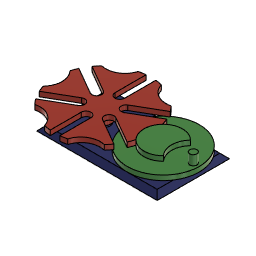
Snowflake (Autodesk Fusion 360 design; units mm, degrees)
Autodesk Fusion 360 part; units mm, degrees
note: some values were not read from the file. Set by a fixed rule: which face or edge a step refers to.
sketch "Base" plane through (0, 0, 0) normal (0, 0, 1) x (1, 0, 0) in component "Base"
  line L0 (125, 75) -> (-125, 75)
  line L1 (-125, 75) -> (-125, -75)
  line L2 (-125, -75) -> (125, -75)
  line L3 (125, -75) -> (125, 75)
  line L4 (125, 75) -> (-125, -75) construction
  line L5 (-125, 75) -> (125, -75) construction
  dimension "d1" = 250
  dimension "d2" = 150
  constraint horizontal L0
  constraint perpendicular L0 L1
  constraint parallel L0 L2
  constraint parallel L1 L3
  constraint coincident L4 origin
  constraint coincident L5 origin
  measures "d1" distance of L1.end L2.end
  measures "d2" distance of L0.end L1.end
extrude "Extrude1" add sketch "Base" along normal blind 10 makes body 1 in component "Base"
sketch "Wheels" plane through (0, 0, 10) normal (0, 0, 1) x (-1, 0, 0) in component "Base"
  line L0 (-125, 75) -> (-125, -75)
  line L1 (-125, -75) -> (125, -75)
  line L2 (125, -75) -> (125, 75)
  line L3 (125, 75) -> (-125, 75)
  line L4 (0, 0) -> (-125, 0) construction
  line L5 (0, 0) -> (125, 0) construction
  line L6 (0, -75) -> (0, 75) construction
  circle A0 centre (-62.5, 0) radius 75
  circle A1 centre (62.5, 0) radius 75
  circle A2 centre (-62.5, 0) radius 15
  circle A3 centre (62.5, 0) radius 15
  dimension "d5" = 150
  dimension "d6" = 30
  dimension "d7" = 30
  constraint coincident L4.start L5.start
  constraint midpoint L0 L4.end
  constraint midpoint L2 L5.end
  constraint midpoint L1 L6.start
  constraint midpoint L3 L6.end
  constraint midpoint L4 A0.centre
  constraint symmetric L6 A0 A1
  constraint concentric A0 A2
  constraint concentric A1 A3
  measures "d5" diameter of A0
  measures "d6" diameter of A2
  measures "d7" diameter of A3
extrude "Extrude2" add sketch "Wheels" along normal blind 20 and the other way blind -10 separate body contours L0 A0 A1 | L0 A0 | A0 A1 makes body 2 in component "Base"
copy_body "CutPasteBodies1" bodies 2 removing the originals makes body 3 in component "Crank"
extrude "Extrude3" add sketch "Wheels" along normal blind 10 contours A2 bodies 1 in component "Base"
extrude "Extrude1'" add sketch "Wheels" along normal blind 30 and the other way blind -20 separate body contours L2 A0 A1 | A0 A1 | L2 A1 makes body 4 in component "Snowflake"
extrude "Extrude4" add sketch "Wheels" along normal blind 20 contours A3 bodies 1 in component "Base"
move_face "OffsetFaces1" offset 25 1 faces at (12.1273, -7.4676, 36.6667) on bodies 4 in component "Snowflake"
move_face "OffsetFaces2" offset 20 1 faces at (-77.4814, -0.7477, 33.3333) on bodies 4 in component "Snowflake"
move_face "OffsetFaces1'" offset 20 1 faces at (47.5186, 0.7477, 26.6667) on bodies 3 in component "Crank"
sketch "Holder" plane through (0, 0, 30) normal (0, 0, -1) x (1, 0, 0) in component "Snowflake"
  circle A0 centre (-62.5, 0) radius 100
  circle A1 centre (-62.5, 0) radius 15
  circle A2 centre (-62.5, 0) radius 17
  dimension "d25" = 30
  dimension "d26" = 2
  constraint concentric A0 A1
  measures "d25" diameter of A1
extrude "Extrude3'" add sketch "Holder" along normal blind 15 contours A2 bodies 4 in component "Snowflake"
sketch "Holder (2)" plane through (0, 0, 20) normal (0, 0, -1) x (1, 0, 0) in component "Crank"
  circle A0 centre (62.5, 0) radius 75
  circle A1 centre (62.5, 0) radius 15
  circle A2 centre (62.5, 0) radius 17
  dimension "d29" = 30
  dimension "d30" = 2
  constraint concentric A0 A1
  measures "d29" diameter of A1
extrude "Extrude1''" add sketch "Holder (2)" along normal blind 8 contours A2 bodies 3 in component "Crank"
move_face "OffsetFaces1''" offset -0.2 1 faces at (-77.4814, 0.7477, 23.3333) on bodies 1 in component "Base"
move_face "OffsetFaces2'" offset -0.2 1 faces at (47.5186, -0.7477, 13.3333) on bodies 1 in component "Base"
sketch "Middle" plane through (0, 0, 30) normal (0, 0, 1) x (-1, 0, 0) in component "Crank"
  circle A0 centre (-62.5, 0) radius 75
  circle A1 centre (-62.5, 0) radius 40
  dimension "d43" = 80
  constraint concentric A0 A1
  measures "d43" diameter of A1
extrude "Extrude2'" add sketch "Middle" along normal blind 10 contours A1 bodies 3 in component "Crank"
extrude "Extrude4'" cut sketch "Middle" along normal blind 10 contours A1 bodies 4 in component "Snowflake"
pattern_circular "C-Pattern1" count 6 over 360 about axis through (-62.5, 0, 40) along (0, 0, 1) of 1 faces at (32.3519, 26.2886, 36.6667) on bodies 4 in component "Snowflake"
sketch "Pin" plane through (0, 0, 30) normal (0, 0, 1) x (-1, 0, 0) in component "Crank"
  circle A0 centre (-62.5, 0) radius 40
  circle A1 centre (-62.5, 0) radius 75
  circle A2 centre (-125, 0) radius 7.5
  dimension "d50" = 15
  measures "d50" diameter of A2
extrude "Extrude3''" add sketch "Pin" along normal blind 20 contours A2 bodies 3 in component "Crank"
sketch "Middle cut" plane through (0, 0, 40) normal (0, 0, 1) x (-1, 0, 0) in component "Crank"
  circle A0 centre (-62.5, 0) radius 40
  arc A1 (-91.0202, -28.0464) -> (-91.1738, 27.8893) centre (-120.1291, -0.1582) ccw
  circle A2 centre (-62.5, 0) radius 40
  constraint concentric A0 A2
  constraint coincident A0 A1.start
  constraint coincident A0 A1.end
sketch "Pin holes" plane through (0, 0, 40) normal (0, 0, 1) x (-1, 0, 0) in component "Snowflake"
  arc A0 (-9.4998, 69.3976) -> (38.3998, 97.0525) centre (0, 108.2532) ccw
  arc A1 (-9.4998, 69.3976) -> (-33.6, 27.6548) centre (62.5, 0) ccw
  arc A2 (-33.6, -27.6548) -> (-33.6, 27.6548) centre (-62.5, 0) ccw
  arc A3 (-33.6, -27.6548) -> (-9.4998, -69.3976) centre (62.5, 0) ccw
  arc A4 (38.3998, -97.0525) -> (-9.4998, -69.3976) centre (0, -108.2532) ccw
  arc A5 (38.3998, -97.0525) -> (86.6002, -97.0525) centre (62.5, 0) ccw
  arc A6 (134.4998, -69.3976) -> (86.6002, -97.0525) centre (125, -108.2532) ccw
  arc A7 (134.4998, -69.3976) -> (158.6, -27.6548) centre (62.5, 0) ccw
  arc A8 (158.6, 27.6548) -> (158.6, -27.6548) centre (187.5, 0) ccw
  arc A9 (158.6, 27.6548) -> (134.4998, 69.3976) centre (62.5, 0) ccw
  arc A10 (86.6002, 97.0525) -> (134.4998, 69.3976) centre (125, 108.2532) ccw
  arc A11 (86.6002, 97.0525) -> (38.3998, 97.0525) centre (62.5, 0) ccw
  circle A12 centre (62.5, 0) radius 25
  line L0 (62.5, -100) -> (62.5, 100) construction
  line L1 (62.5, -100) -> (72.5, -100) construction
  line L2 (62.5, -100) -> (52.5, -100) construction
  line L3 (72.5, -100) -> (72.5, -35)
  line L4 (52.5, -100) -> (52.5, -35)
  line L5 (62.5, -25) -> (62.5, -25)
  arc A13 (72.5, -35) -> (62.5, -25) centre (62.5, -35) ccw
  arc A14 (62.5, -25) -> (52.5, -35) centre (62.5, -35) ccw
  line L6 (144.1025, -58.6603) -> (87.8109, -26.1603)
  line L7 (154.1025, -41.3397) -> (97.8109, -8.8397)
  arc A15 (97.8109, -8.8397) -> (84.1506, -12.5) centre (92.8109, -17.5) ccw
  arc A16 (84.1506, -12.5) -> (87.8109, -26.1603) centre (92.8109, -17.5) ccw
  line L8 (149.1025, -50) -> (144.1025, -58.6603) construction
  line L9 (149.1025, -50) -> (154.1025, -41.3397) construction
  line L10 (154.1025, 41.3397) -> (97.8109, 8.8397)
  line L11 (144.1025, 58.6603) -> (87.8109, 26.1603)
  arc A17 (87.8109, 26.1603) -> (84.1506, 12.5) centre (92.8109, 17.5) ccw
  arc A18 (84.1506, 12.5) -> (97.8109, 8.8397) centre (92.8109, 17.5) ccw
  line L12 (149.1025, 50) -> (154.1025, 41.3397) construction
  line L13 (149.1025, 50) -> (144.1025, 58.6603) construction
  line L14 (72.5, 100) -> (72.5, 35)
  line L15 (52.5, 100) -> (52.5, 35)
  arc A19 (52.5, 35) -> (62.5, 25) centre (62.5, 35) ccw
  arc A20 (62.5, 25) -> (72.5, 35) centre (62.5, 35) ccw
  line L16 (62.5, 100) -> (72.5, 100) construction
  line L17 (62.5, 100) -> (52.5, 100) construction
  line L18 (-19.1025, 58.6603) -> (37.1891, 26.1603)
  line L19 (-29.1025, 41.3397) -> (27.1891, 8.8397)
  arc A21 (27.1891, 8.8397) -> (40.8494, 12.5) centre (32.1891, 17.5) ccw
  arc A22 (40.8494, 12.5) -> (37.1891, 26.1603) centre (32.1891, 17.5) ccw
  line L20 (-24.1025, 50) -> (-19.1025, 58.6603) construction
  line L21 (-24.1025, 50) -> (-29.1025, 41.3397) construction
  line L22 (-29.1025, -41.3397) -> (27.1891, -8.8397)
  line L23 (-19.1025, -58.6603) -> (37.1891, -26.1603)
  arc A23 (37.1891, -26.1603) -> (40.8494, -12.5) centre (32.1891, -17.5) ccw
  arc A24 (40.8494, -12.5) -> (27.1891, -8.8397) centre (32.1891, -17.5) ccw
  line L24 (-24.1025, -50) -> (-29.1025, -41.3397) construction
  line L25 (-24.1025, -50) -> (-19.1025, -58.6603) construction
  dimension "d56" = 50
  dimension "d59" = 10
  dimension "d60" = 10
  dimension "d61" = 10
  dimension "d63" = 360
  constraint concentric A1 A12
  constraint midpoint A5 L0.start
  constraint midpoint A11 L0.end
  constraint perpendicular L0 L1
  constraint perpendicular L0 L2
  constraint perpendicular L1 L3
  constraint perpendicular L2 L4
  constraint tangent L3 A13
  constraint tangent L4 A14
  constraint equal A13 A14
  measures "d56" diameter of A12
  measures "d59" distance of L0.start L1.end
  measures "d60" distance of L0.start L2.end
  measures "d61" radius of A13
extrude "Extrude5" cut sketch "Pin holes" against normal blind 10 contours A1 L18 L19 A21 A22 | A11 L14 L15 A19 A20 | A3 L22 L23 A23 A24 | A9 L10 L11 A17 A18 | A5 L3 L4 A13 A14 | A7 L6 L7 A15 A16 bodies 4 in component "Snowflake"
extrude "Extrude5'" cut sketch "Middle cut" against normal blind 10 contours A0 A1 A2 picked at (-94.6295, -4.7565) bodies 3 in component "Crank"
chamfer "Chamfer1" distance 10 angle 45 4 edges at (0, -75, 10) (125, 0, 10) (0, 75, 10) (-125, 0, 10) on bodies 1 in component "Base"
extrude "Extrude4''" [suppressed] in component "Crank"
component "Base" placed x (1, 0, 0) y (0, 1, 0) z (0, 0, 1) at (0, 0, 0)
component "Snowflake" placed x (1, 0, 0) y (0, 1, 0) z (0, 0, 1) at (0, 0, 0)
component "Crank" placed x (-0.5, 0.866025, 0) y (-0.866025, -0.5, 0) z (0, 0, 1) at (93.75, -54.1266, 0)
named bodies: "Base", "Crank", "Snowflake"
